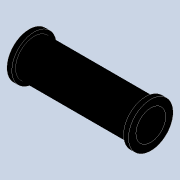
# Autodesk Inventor part: Filament Spool Holder
Saved by Autodesk Inventor 2022 (Build 260153000, 153)
## iProperties
Created: 2022-02-06
Part Number: Filament Spool Holder
Material: Generic
Document SubType Name: Modeling
Designer: Coy
Density: 1 g/cm^3
Appearance: Anodized - Black
Author: Coy
Autodesk Inventor part; units mm, degrees
ref_plane "YZ Plane" through (0, 0, 0) normal (1, 0, 0) x (0, 1, 0)
ref_plane "XZ Plane" through (0, 0, 0) normal (0, 1, 0) x (-1, 0, 0)
ref_plane "XY Plane" through (0, 0, 0) normal (0, 0, 1) x (1, 0, 0)
sketch "Sketch1" plane through (0, 0, 0) normal (0, 0, 1) x (1, 0, 0)
  line L0 (0, 3) -> (0, 18)
  line L1 (0, 18) -> (4, 18)
  line L2 (4, 18) -> (4, 15)
  line L3 (4, 15) -> (94, 15)
  line L4 (94, 15) -> (94, 18)
  line L5 (94, 18) -> (98, 18)
  line L6 (98, 18) -> (98, 12)
  line L7 (98, 12) -> (3, 12)
  line L8 (3, 12) -> (3, 3)
  line L9 (3, 0) -> (0, 0) construction
  line L10 (0, 3) -> (3, 3)
  dimension "d0" = 18
  dimension "d1" = 4
  dimension "d2" = 3
  dimension "d3" = 90
  dimension "d4" = 4
  dimension "d5" = 6
  dimension "d6" = 95
  dimension "d7" = 3
  constraints: 22 end point, 9 perpendicular, 2 point on line, 1 vertical
  measures "d0" distance of L9.end L0.end
  measures "d1" distance of L0.end L1.end
  measures "d2" distance of L1.end L2.end
  measures "d3" distance of L2.end L3.end
  measures "d4" distance of L4.end L5.end
  measures "d5" distance of L5.end L6.end
  measures "d6" distance of L6.end L7.end
  measures "d7" distance between parallel lines of L9 L10
revolve "Revolution1" add sketch "Sketch1" angle 360 about axis through (3, 0, 0) along (-1, 0, 0)
body "Solid1"
